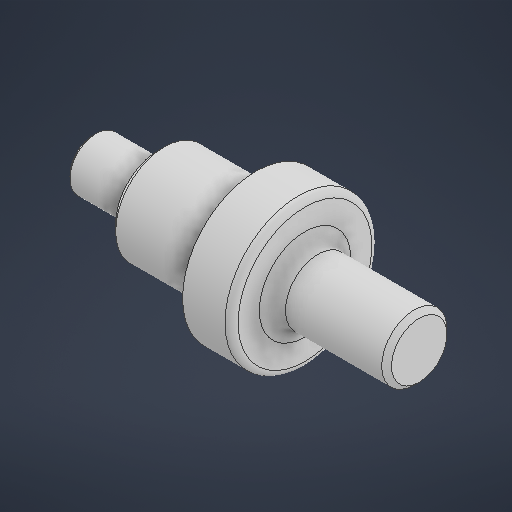
# Autodesk Inventor part: Part13
Saved by Autodesk Inventor 2026 (Build 300175050, 175E)
## iProperties
Created: 2026-03-26
Part Number: Part13
Material: Generic
Document SubType Name: Modeling
Designer: Administrator
Density: 1 g/cm^3
Appearance: Default
Author: Administrator
Autodesk Inventor part; units mm, degrees
ref_plane "YZ Plane" through (0, 0, 0) normal (1, 0, 0) x (0, 1, 0)
ref_plane "XZ Plane" through (0, 0, 0) normal (0, 1, 0) x (-1, 0, 0)
ref_plane "XY Plane" through (0, 0, 0) normal (0, 0, 1) x (1, 0, 0)
sketch "Sketch1" plane through (0, 0, 0) normal (0, 0, 1) x (1, 0, 0)
  line L0 (100, 10) -> (100, 0)
  line L1 (50.009, 15) -> (20.009, 15)
  line L2 (20.009, 15) -> (20.009, 15)
  line L3 (20.009, 15) -> (20, 15)
  line L4 (20, 15) -> (20, 8)
  line L5 (20, 8) -> (0, 8)
  line L6 (0, 8) -> (0, 0)
  line L7 (50.009, 15) -> (50.009, 22.5)
  line L8 (50.009, 22.5) -> (65.009, 22.5)
  line L9 (65.009, 22.5) -> (65.009, 10)
  line L10 (65.009, 10) -> (100, 10)
  line L11 (100, 10) -> (100, 10)
  line L12 (0, 0) -> (100, 0)
  dimension "d0" = 100
  dimension "d5" = 20
  dimension "d6" = 30
  dimension "d7" = 20
  dimension "d8" = 45
  dimension "d9" = 30
  dimension "d10" = 16
  dimension "d11" = 15
  constraints: 26 end point, 8 perpendicular, 2 horizontal, 1 vertical
  measures "d0" distance of L6.end L0.end
  measures "d5" distance of L4.end L5.end
  measures "d6" distance of L1.start L1.end
  measures "d7" diameter of L10 L12
  measures "d8" diameter of L8 L12
  measures "d9" diameter of L1 L12
  measures "d10" diameter of L5 L12
  measures "d11" distance of L7.end L8.end
revolve "Revolution1" add sketch "Sketch1" angle 360 mid plane about axis through (0, 0, 0) along (1, 0, 0)
chamfer "Chamfer1" distance 1.5 angle 45 1 edges at (100, 10, 0)
fillet "Fillet1" radius 4 1 edges at (65.009, 10, 0)
fillet "Fillet2" radius 2 1 edges at (65.009, 22.5, 0)
chamfer "Chamfer2" distance 2 angle 45 1 edges at (20, 15, 0)
chamfer "Chamfer3" distance 1 angle 45 1 edges at (0, 8, 0)
body "Solid1"
